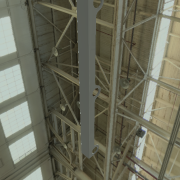
# Autodesk Inventor part: Randschiene 7L
Saved by Autodesk Inventor 2015 (Build 190159000, 159)
## iProperties
Created: 2017-04-11
Part Number: Randschiene 7L
Material: Generic
Document SubType Name: Modeling
Designer: Seelenernter
Density: 1 g/cm^3
Appearance: Galvanisiert
Author: Seelenernter
Autodesk Inventor part; units mm, degrees
sketch "Skizze1" plane through (0, 0, 0) normal (0, 0, 1) x (1, 0, 0)
  line L0 (0, 60) -> (0, -10) projected
  line L1 (-56, 0) -> (56, 0) projected
  line L2 (-56, 0) -> (56, 0) projected
  line L3 (0, -10) -> (0, 60) projected
  line L4 (-40, 0) -> (40, 0)
  line L5 (-40, 0) -> (-40, 50)
  line L6 (40, 0) -> (40, 50)
  line L7 (-35, 50) -> (-35, 5)
  line L8 (-35, 5) -> (35, 5)
  line L9 (35, 5) -> (35, 50)
  line L10 (-40, 50) -> (-35, 50)
  line L11 (40, 50) -> (35, 50)
  point P0 (0, 0)
  point P1 (0, 0)
  dimension "d0" = 80
  dimension "d1" = 50
  dimension "d2" = 50
  dimension "d4" = 5
  constraints: 16 end point, 2 point on line, 2 vertical, 1 coincident, 1 collinear, 1 horizontal, 1 midpoint, 2 other
  measures "d0" distance between parallel lines of L6 L5
  measures "d1" distance of L4.end L6.end
  measures "d2" distance of L4.start L5.end
  measures "d4" distance between parallel lines of L5 L7
extrude "Extrusion1" add sketch "Skizze1" along normal blind 585
fillet "Rundung1" radius 2.5 2 edges at (-35, 5, 292.5) (35, 5, 292.5)
fillet "Rundung1" radius 5 2 edges at (40, 0, 292.5) (-40, 0, 292.5)
sketch "Skizze2" plane through (40, 50, 585) normal (1, 0, 0) x (0, 0, -1)
  line L0 (585, -45) -> (0, -45) projected
  line L1 (585, -45) -> (585, 0) projected
  line L2 (585, 0) -> (0, 0) projected
  line L3 (0, -45) -> (0, 0) projected
  line L4 (0, -45) -> (0, -50) projected
  line L5 (0, -50) -> (585, -50) projected
  line L6 (585, -50) -> (585, -45) projected
  line L7 (585, -45) -> (0, -45) projected
  arc A0 (85, 7.5) -> (0, 7.5) centre (42.5, 7.5) ccw
  line L8 (0, 7.5) -> (0, 0)
  line L9 (85, 7.5) -> (85, 0)
  point P0 (585, -50)
  dimension "d9" = 85
  dimension "d10" = 100
  dimension "d11" = 42.5
  constraints: 4 end point, 2 point on circle, 1 centre point, 1 perpendicular, 1 point on line, 1 tangent, 1 vertical
  measures "d9" diameter of A0
  measures "d11" distance from line of L3 A0.centre
extrude "Extrusion2" add sketch "Skizze2" against normal blind 5 contours L8 A0 L9 L2
sketch "Skizze3" plane through (40, 5, 0) normal (1, 0, 0) x (0, 0, -1)
  line L0 (0, 0) -> (-585, 0) projected
  line L1 (0, 0) -> (0, 45) projected
  line L2 (0, 45) -> (-500, 45) projected
  line L3 (-500, 45) -> (-500, 52.5) projected
  arc A0 (-500, 52.5) -> (-585, 52.5) centre (-542.5, 52.5) ccw projected
  line L4 (-585, 0) -> (-585, 52.5) projected
  circle A1 centre (-542.5, 52.5) radius 27.5
  point P0 (0, -5)
  dimension "d14" = 55
  constraints: 1 centre point, 1 coincident
  measures "d14" diameter of A1
extrude "Extrusion3" cut sketch "Skizze3" against normal blind 5 contours A1
ref_plane "Arbeitsebene1" through (40, 5, 292.5) normal (0, 0, 1) x (1, 0, 0)
ref_plane "Arbeitsebene2" through (0, 0, 0) normal (1, 0, 0) x (0, 1, 0)
mirror "Spiegeln1" about plane through (40, 5, 292.5) normal (0, 0, 1) of "Extrusion2", "Extrusion3"
mirror "Spiegeln2" about plane through (0, 0, 0) normal (1, 0, 0) of "Extrusion2", "Extrusion3", "Spiegeln1"
fillet "Rundung2" radius 30 4 edges at (37.5, 50, 500) (-37.5, 50, 500) (-37.5, 50, 85) (37.5, 50, 85)
ref_plane "Arbeitsebene4" through (40, 57.5, 542.5) normal (0, 0, 1) x (-1, 0, 0)
mirror "Spiegeln3" about plane through (40, 57.5, 542.5) normal (0, 0, 1) of "Extrusion1", "Rundung1", "Rundung2", "Extrusion2", "Extrusion3", "Spiegeln1", "Spiegeln2"
